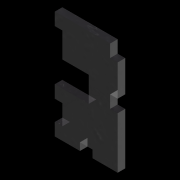
# Autodesk Inventor part: SideLeftTopNM
Saved by Autodesk Inventor 2019 (Build 230136000, 136)
## iProperties
Created: 2019-05-08
Part Number: SideLeftTopNM
Material: Acrylic, Clear
Document SubType Name: Modeling
Designer: super pig
Density: 1.19 g/cm^3
Appearance: Transparent - Clear
Mass: 2.76675 g
Surface Area: 20.6912 cm^2
Volume: 2.325 cm^3
Name: Left Side Top Cover
Author: super pig
Autodesk Inventor part; units mm, degrees
ref_plane "YZ Plane" through (0, 0, 0) normal (1, 0, 0) x (0, 1, 0)
ref_plane "XZ Plane" through (0, 0, 0) normal (0, 1, 0) x (-1, 0, 0)
ref_plane "XY Plane" through (0, 0, 0) normal (0, 0, 1) x (1, 0, 0)
sketch "Sketch1" plane through (0, 0, 0) normal (0, 0, 1) x (1, 0, 0)
  line L0 (-3, 22.15) -> (-3, 34.65) projected
  line L1 (-3, 17.15) -> (-3, 22.15) projected
  line L2 (-3, -3.35) -> (-3, 17.15) projected
  line L3 (0, -3.35) -> (-3, -3.35) projected
  line L4 (0, 17.15) -> (0, -3.35) projected
  line L5 (0, 17.15) -> (-3, 17.15) projected
  line L6 (-3, 34.65) -> (-3, 39.65) projected
  line L7 (-3, -3.35) -> (-22, -3.35)
  line L8 (-22, -3.35) -> (-22, 39.65)
  line L9 (-22, 39.65) -> (-3, 39.65)
  line L10 (-22, 39.65) -> (-25, 39.65)
  line L11 (-25, 39.65) -> (-25, 34.65)
  line L12 (-25, 34.65) -> (-22, 34.65)
  line L13 (-22, 34.65) -> (-22, 39.65)
  line L14 (-22, 24.65) -> (-11.5, 24.65)
  line L15 (-11.5, 24.65) -> (-11.5, 14.65)
  line L16 (-11.5, 14.65) -> (-22, 14.65)
  line L17 (-22, 14.65) -> (-25, 14.65)
  line L18 (-25, 14.65) -> (-25, 9.65)
  line L19 (-25, 9.65) -> (-22, 9.65)
  line L20 (-22, 9.65) -> (-22, 14.65)
  line L21 (-22, -3.35) -> (-25, -3.35)
  line L22 (-25, -3.35) -> (-25, 1.65)
  line L23 (-25, 1.65) -> (-22, 1.65)
  line L24 (-22, 1.65) -> (-22, -3.35)
  line L25 (-15, -3.35) -> (-10, -3.35)
  line L26 (-10, -3.35) -> (-10, -0.35)
  line L27 (-10, -0.35) -> (-15, -0.35)
  line L28 (-15, -0.35) -> (-15, -3.35)
  line L29 (-3, 22.15) -> (-3, 34.65) projected
  line L30 (0, 22.15) -> (-3, 22.15) projected
  line L31 (0, 34.65) -> (0, 22.15) projected
  line L32 (0, 34.65) -> (-3, 34.65) projected
  point P0 (-11.5, 19.65)
  point P1 (-3, 19.65)
  point P2 (-12.5, -3.35)
  dimension "d1" = 19
  dimension "d2" = 3
  dimension "d3" = 5
  dimension "d4" = 10
  dimension "d8" = 3
  dimension "d9" = 5
  dimension "d10" = 3
  dimension "d11" = 5
  dimension "d12" = 5
  dimension "d13" = 3
  dimension "d16" = 8.5
  constraints: 44 end point, 9 parallel, 7 perpendicular, 6 horizontal, 4 midpoint, 3 point on line, 1 horizontal alignment
  measures "d1" distance of L2.start L7.end
  measures "d2" distance of L12.end L11.end
  measures "d3" distance of L11.end L10.end
  measures "d4" distance between parallel lines of L14 L16
  measures "d8" distance of L19.end L18.end
  measures "d9" distance of L18.end L17.end
  measures "d10" distance of L22.end L23.end
  measures "d11" distance of L21.end L22.end
  measures "d12" distance of L27.end L26.end
  measures "d13" distance of L26.end L25.end
  measures "d16" distance between parallel lines of L1 L15
extrude "Extrusion1" add sketch "Sketch1" along normal blind 3 contours L1 L2 L7 L26 L27 L28 L8 L16 L15 L14 L9 L6 L0 | L0 L32 L31 L30 | L5 L4 L3 L2 | L8 L12 L11 L10 | L21 L22 L23 L8 | L8 L19 L18 L17
body "Solid1"
